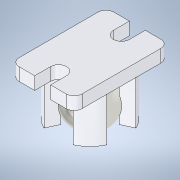
# Autodesk Inventor part: Roue_libre
Saved by Autodesk Inventor 2022 (Build 260153000, 153)
## iProperties
Created: 2020-11-24
Part Number: Roue_libre
Material: Générique
Document SubType Name: Modeling
Designer: utilisateur
Density: 1 g/cm^3
Appearance: Par défaut
Author: utilisateur
Autodesk Inventor part; units mm, degrees
ref_plane "YZ Plane" through (0, 0, 0) normal (1, 0, 0) x (0, 1, 0)
ref_plane "XZ Plane" through (0, 0, 0) normal (0, 1, 0) x (-1, 0, 0)
sketch "Esquisse1" plane through (0, 0, 0) normal (1, 0, 0) x (0, 1, 0)
  line L0 (11.9, 7.9) -> (-11.9, 7.9)
  line L1 (-11.9, 7.9) -> (-11.9, -7.9)
  line L2 (-11.9, -7.9) -> (11.9, -7.9)
  line L3 (11.9, -7.9) -> (11.9, 7.9)
  point P0 (0, 0)
  point P1 (11.9, 0)
  point P2 (0, -7.9)
  dimension "d0" = 23.8
  dimension "d3" = 15.8
  constraints: 8 end point, 2 midpoint, 2 perpendicular, 1 horizontal, 1 horizontal alignment, 1 vertical, 1 vertical alignment
  measures "d0" distance of L1.end L2.end
  measures "d3" distance of L2.end L0.start
extrude "Extrusion1" add sketch "Esquisse1" along normal mid plane 3.2
sketch "Esquisse2" plane through (1.6, 0, 0) normal (1, 0, 0) x (0, 0, -1)
  circle A0 centre (0, 0) radius 8.7
  line L0 (7.9, -11.9) -> (7.9, 11.9) projected
  line L1 (7.9, 3.6442) -> (0, 0)
  line L2 (0, 0) -> (7.9, -3.6442)
  line L3 (0, 0) -> (-7.9, -3.6442)
  line L4 (-7.9, 11.9) -> (-7.9, -11.9) projected
  line L5 (0, 0) -> (-7.9, 3.6442)
  line L6 (0, 0) -> (3.6423, -7.9008)
  line L7 (0, 0) -> (-3.6423, -7.9008)
  line L8 (0, 0) -> (3.6423, 7.9008)
  line L9 (0, 0) -> (-3.6423, 7.9008)
  line L10 (3.6423, 7.9008) -> (-3.6423, 7.9008) construction
  line L11 (3.6423, -7.9008) -> (-3.6423, -7.9008) construction
  line L12 (0, -7.9008) -> (0, 7.9008) construction
  circle A1 centre (0, 0) radius 5.5
  point P0 (2.3026, 4.9948)
  point P1 (4.9943, 2.3038)
  point P2 (-4.9943, 2.3038)
  point P3 (-2.3026, 4.9948)
  point P4 (-2.3026, -4.9948)
  point P5 (-4.9943, -2.3038)
  point P6 (4.9943, -2.3038)
  point P7 (2.3026, -4.9948)
  dimension "d4" = 17.4
  dimension "d7" = 49.5
  dimension "d8" = 49.5
  dimension "d9" = 11
  constraints: 22 end point, 4 point on line, 2 coincident, 2 horizontal, 2 midpoint, 1 centre point, 10 other
  measures "d7" angle of L7 L6
  measures "d8" angle of L9 L8
  measures "d9" diameter of A1
extrude "Extrusion3" add sketch "Esquisse2" along normal blind 11 contours L1 A1 L8 A0 | A0 L6 A1 L2 | L9 A1 L5 A0 | A0 L3 A1 L7
sketch "Esquisse3" plane through (1.6, 0, 0) normal (1, 0, 0) x (0, 0, -1)
  line L0 (0, -7.9) -> (0, -17.3183) construction
  line L1 (-2, -7.9) -> (-2, -17.3183)
  line L2 (2, -17.3183) -> (2, -7.9)
  arc A0 (2, -7.9) -> (-2, -7.9) centre (0, -7.9) ccw
  arc A1 (-2, -17.3183) -> (2, -17.3183) centre (0, -17.3183) ccw
  line L3 (-7.9, -11.9) -> (7.9, -11.9) projected
  line L4 (0, -25.5619) -> (0, 18.1437) projected
  point P0 (0, 0)
  point P1 (0, -12.6091)
  point P2 (2, -11.9)
  point P3 (-2, -11.9)
  dimension "d12" = 4
  dimension "d13" = 4
  constraints: 8 end point, 4 point on circle, 4 tangent, 2 centre point, 1 collinear, 1 midpoint, 1 parallel, 1 vertical
  measures "d12" distance between parallel lines of L1 L2
  measures "d13" distance from line of L3 L0.start
extrude "Extrusion4" cut sketch "Esquisse3" against normal blind 11 contours A0 L4 L3 L1 | A0 L2 L3 L4
mirror "Symétrie1" about plane through (0, 0, 0) normal (0, 1, 0) of "Extrusion4"
sketch "Esquisse4" plane through (0, 0, 0) normal (0, 0, 1) x (1, 0, 0)
  circle A0 centre (8.5, 0) radius 6
  line L0 (14.5, 0) -> (-1.6, 0)
  line L1 (-1.6, -11.9) -> (-1.6, 11.9) projected
  point P0 (0, 0)
  point P1 (2.5, 0)
  dimension "d16" = 12
  dimension "d17" = 16.1
  constraints: 2 end point, 1 midpoint, 3 other
  measures "d17" distance of L0.start L0.end
revolve "Révolution1" add sketch "Esquisse4" angle 360 about axis through (14.5, 0, 0) along (-1, 0, 0) picked at (6.7291, -0.9294) contours A0 L0
fillet "Congé1" radius 2 4 edges at (0, 11.9, 7.9) (0, 11.9, -7.9) (0, -11.9, -7.9) (0, -11.9, 7.9)
ref_plane "Plan de construction1" through (14.5, 0, 0) normal (1, 0, 0) x (0, 1, 0)
